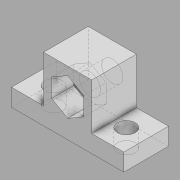
# Autodesk Inventor part: y_axis_lead_screw_insert
Saved by Autodesk Inventor 2020 (Build 240168000, 168)
## iProperties
Created: 2021-04-21
Part Number: y_axis_lead_screw_insert
Material: Generic
Document SubType Name: Modeling
Designer: griss
Density: 1 g/cm^3
Appearance: Default
Author: griss
Autodesk Inventor part; units mm, degrees
ref_plane "YZ Plane" through (0, 0, 0) normal (1, 0, 0) x (0, 1, 0)
ref_plane "XZ Plane" through (0, 0, 0) normal (0, 1, 0) x (-1, 0, 0)
ref_plane "XY Plane" through (0, 0, 0) normal (0, 0, 1) x (1, 0, 0)
sketch "Sketch1" plane through (0, 0, 0) normal (0, 0, 1) x (1, 0, 0)
  line L0 (0, 0) -> (-25.5293, 0)
  line L1 (-25.5293, 0) -> (-25.5293, 7.9022)
  line L2 (-25.5293, 7.9022) -> (-10.9446, 7.9022)
  line L3 (-10.9446, 7.9022) -> (-10.9446, 28.9877)
  line L4 (0, -5.7975) -> (0, 34.7852) projected
  line L5 (0, 0) -> (25.5293, 0)
  line L6 (25.5293, 0) -> (25.5293, 7.9022)
  line L7 (25.5293, 7.9022) -> (10.9446, 7.9022)
  line L8 (10.9446, 7.9022) -> (10.9446, 28.9877)
  line L9 (10.9446, 28.9877) -> (-10.9446, 28.9877)
  constraints: 18 end point, 4 symmetric about line, 3 perpendicular, 1 horizontal
extrude "Extrusion1" add sketch "Sketch1" along normal mid plane 20.32
sketch "Sketch2" plane through (0, 0, 10.16) normal (0, 0, 1) x (1, 0, 0)
  line L0 (-10.9446, 7.9022) -> (-25.5293, 7.9022) projected
  line L1 (-25.5293, 7.9022) -> (-25.5293, 0) projected
  line L2 (-25.5293, 0) -> (25.5293, 0) projected
  line L3 (25.5293, 0) -> (25.5293, 7.9022) projected
  line L4 (25.5293, 7.9022) -> (10.9446, 7.9022) projected
  line L5 (10.9446, 7.9022) -> (10.9446, 28.9877) projected
  line L6 (10.9446, 28.9877) -> (-10.9446, 28.9877) projected
  line L7 (-10.9446, 28.9877) -> (-10.9446, 7.9022) projected
  line L8 (0, -6.2231) -> (0, 37.3386) projected
  line L9 (0, 25.2482) -> (7.2771, 21.0468)
  line L10 (7.2771, 21.0468) -> (7.2771, 12.6439)
  line L11 (7.2771, 12.6439) -> (0, 8.4425)
  line L12 (0, 8.4425) -> (-7.2771, 12.6439)
  line L13 (-7.2771, 12.6439) -> (-7.2771, 21.0468)
  line L14 (-7.2771, 21.0468) -> (0, 25.2482)
  circle A0 centre (0, 16.8453) radius 4.8006
  point P0 (0, 0)
  dimension "d5" = 14.5542
  dimension "d6" = 9.6012
  constraints: 12 end point, 2 point on line, 1 centre point, 1 coincident, 13 other
  measures "d5" distance between parallel lines of L10 L13
  measures "d6" diameter of A0
extrude "Extrusion2" cut sketch "Sketch2" against normal through all contours A0 L8 | L8 A0
extrude "Extrusion3" cut sketch "Sketch2" against normal blind 10.16 contours L9 L10 L11 L8 A0 | L8 A0 L12 L13 L14
sketch "Sketch3" plane through (-25.5293, 7.9022, 10.16) normal (0, 1, 0) x (1, 0, 0)
  line L0 (0, 20.32) -> (0, 0) projected
  line L1 (14.5848, 0) -> (0, 0) projected
  line L2 (14.5848, 20.32) -> (14.5848, 0) projected
  line L3 (0, 20.32) -> (14.5848, 20.32) projected
  line L4 (36.4739, 20.32) -> (36.4739, 0) projected
  line L5 (51.0586, 0) -> (36.4739, 0) projected
  line L6 (51.0586, 20.32) -> (51.0586, 0) projected
  line L7 (36.4739, 20.32) -> (51.0586, 20.32) projected
  circle A0 centre (9.0193, 10.16) radius 4.0005
  line L8 (14.5848, 20.32) -> (14.5848, 0) projected
  line L9 (36.4739, 0) -> (14.5848, 0) projected
  line L10 (36.4739, 20.32) -> (36.4739, 0) projected
  line L11 (14.5848, 20.32) -> (36.4739, 20.32) projected
  line L12 (25.5293, 24.384) -> (25.5293, -4.064) projected
  circle A1 centre (42.0393, 10.16) radius 4.0005
  point P0 (25.5293, 10.16)
  point P1 (0, 10.16)
  dimension "d11" = 8.001
  dimension "d15" = 33.02
  constraints: 2 centre point, 1 horizontal alignment, 1 midpoint, 1 symmetric about line, 1 other
  measures "d11" diameter of A0
  measures "d15" distance of A1.centre A0.centre
extrude "Extrusion4" cut sketch "Sketch3" against normal through all contours A0 | A1
body "Solid1"
